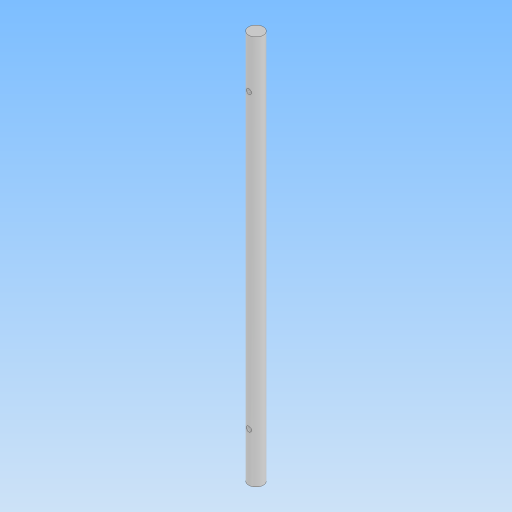
# Autodesk Inventor part: Stange test
Saved by Autodesk Inventor 2024.4 (Build 284460000, 460)
## iProperties
Created: 2026-01-19
Part Number: Stange test
Material: Generisch
Document SubType Name: Modeling
Designer: lucas
Mass: 70.1046 g
Surface Area: 195.808 cm^2
Volume: 70.1046 cm^3
Density: 1 g/cm^3
Appearance: Vorgabe
Masse[kg]: 0,070 kg
Autodesk Inventor part; units mm, degrees
ref_plane "YZ Plane" through (0, 0, 0) normal (1, 0, 0) x (0, 1, 0)
ref_plane "XZ Plane" through (0, 0, 0) normal (0, 1, 0) x (-1, 0, 0)
ref_plane "XY Plane" through (0, 0, 0) normal (0, 0, 1) x (1, 0, 0)
sketch "Skizze1" plane through (0, 0, 0) normal (0, 0, 1) x (1, 0, 0)
  circle A0 centre (0, 0) radius 7.5
  dimension "d0" = 15
  constraints: 1 centre point, 1 coincident
  measures "d0" diameter of A0
extrude "Extrusion1" add sketch "Skizze1" along normal mid plane 400
sketch "Skizze3" plane through (0, 0, 0) normal (0, 1, 0) x (-1, 0, 0)
  circle A0 centre (0, 150) radius 2.5
  circle A1 centre (0, -150) radius 2.5
  point P0 (0, 0)
  dimension "d7" = 5
  dimension "d8" = 5
  constraints: 2 centre point
  measures "d7" diameter of A0
  measures "d8" diameter of A1
extrude "Extrusion3" cut sketch "Skizze3" along normal mid plane 15
